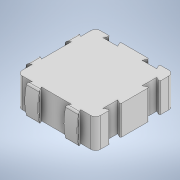
# Autodesk Inventor part: 2x2Base
Saved by Autodesk Inventor 2022.3 (Build 263350030, 350C)
## iProperties
Created: 2022-08-21
Part Number: 2x2Base
Material: Generic
Document SubType Name: Modeling
Designer: yiunf
Density: 1 g/cm^3
Appearance: Default
Author: yiunf
Autodesk Inventor part; units mm, degrees
ref_plane "YZ Plane" through (0, 0, 0) normal (1, 0, 0) x (0, 1, 0)
sketch "Sketch2" plane through (0, 0, 0) normal (0, 1, 0) x (-1, 0, 0)
  line L0 (-40, -40) -> (40, -40)
  line L1 (40, -40) -> (40, 40)
  line L2 (40, 40) -> (-40, 40)
  line L3 (-40, 40) -> (-40, -40)
  line L4 (-40, -40) -> (40, 40) construction
  line L5 (40, -40) -> (-40, 40) construction
  line L6 (0, 40) -> (40, 40)
  line L7 (20, 40) -> (20, 45)
  line L8 (20, 45) -> (27.5, 45)
  line L9 (20, 40) -> (25, 40)
  line L10 (25, 40) -> (27.5, 45)
  line L11 (20, 45) -> (12.5, 45)
  line L12 (20, 40) -> (15, 40)
  line L13 (15, 40) -> (12.5, 45)
  line L14 (20, 44.75) -> (27.0955, 44.75)
  line L15 (27.0955, 44.75) -> (24.8455, 40.25)
  line L16 (24.8455, 40.25) -> (20, 40.25)
  line L17 (20, 44.75) -> (12.9045, 44.75)
  line L18 (12.9045, 44.75) -> (15.1545, 40.25)
  line L19 (15.1545, 40.25) -> (20, 40.25)
  line L20 (20, 44.75) -> (20, 43.75)
  line L21 (20, 43.75) -> (26.875, 43.75)
  line L22 (20, 43.75) -> (13.125, 43.75)
  line L23 (40, 20) -> (45, 20)
  line L24 (45, 20) -> (45, 27.5)
  line L25 (40, 20) -> (40, 25)
  line L26 (40, 25) -> (45, 27.5)
  line L27 (40, 20) -> (40, 15)
  line L28 (40, 15) -> (45, 12.5)
  line L29 (45, 20) -> (45, 12.5)
  line L30 (44.75, 20) -> (44.75, 27.0955)
  line L31 (44.75, 27.0955) -> (40.25, 24.8455)
  line L32 (40.25, 24.8455) -> (40.25, 20)
  line L33 (44.75, 20) -> (44.75, 12.9045)
  line L34 (44.75, 12.9045) -> (40.25, 15.1545)
  line L35 (40.25, 15.1545) -> (40.25, 20)
  line L36 (44.75, 20) -> (43.75, 20)
  line L37 (43.75, 20) -> (43.75, 26.875)
  line L38 (43.75, 20) -> (43.75, 13.125)
  line L39 (-20, 40) -> (-20, 45)
  line L40 (-20, 44.75) -> (-20, 43.75)
  line L41 (-24.8455, 40.25) -> (-20, 40.25)
  line L42 (-20, 40) -> (-25, 40)
  line L43 (-27.0955, 44.75) -> (-24.8455, 40.25)
  line L44 (-25, 40) -> (-27.5, 45)
  line L45 (-20, 43.75) -> (-26.875, 43.75)
  line L46 (-20, 45) -> (-27.5, 45)
  line L47 (-20, 44.75) -> (-27.0955, 44.75)
  line L48 (-15.1545, 40.25) -> (-20, 40.25)
  line L49 (-20, 40) -> (-15, 40)
  line L50 (-20, 43.75) -> (-13.125, 43.75)
  line L51 (-20, 44.75) -> (-12.9045, 44.75)
  line L52 (-20, 45) -> (-12.5, 45)
  line L53 (-12.9045, 44.75) -> (-15.1545, 40.25)
  line L54 (-15, 40) -> (-12.5, 45)
  line L55 (40, -20) -> (40, -15)
  line L56 (44.75, -12.9045) -> (40.25, -15.1545)
  line L57 (40, -15) -> (45, -12.5)
  line L58 (43.75, -20) -> (43.75, -13.125)
  line L59 (44.75, -20) -> (44.75, -12.9045)
  line L60 (45, -20) -> (45, -12.5)
  line L61 (40.25, -15.1545) -> (40.25, -20)
  line L62 (40, -20) -> (45, -20)
  line L63 (40.25, -24.8455) -> (40.25, -20)
  line L64 (40, -20) -> (40, -25)
  line L65 (44.75, -27.0955) -> (40.25, -24.8455)
  line L66 (40, -25) -> (45, -27.5)
  line L67 (43.75, -20) -> (43.75, -26.875)
  line L68 (44.75, -20) -> (44.75, -27.0955)
  line L69 (45, -20) -> (45, -27.5)
  line L70 (44.75, -20) -> (43.75, -20)
  line L71 (20, -35) -> (27.5, -35)
  line L72 (25, -40) -> (27.5, -35)
  line L73 (20, -35) -> (12.5, -35)
  line L74 (15, -40) -> (12.5, -35)
  line L75 (-15, -40) -> (-12.5, -35)
  line L76 (-20, -35) -> (-12.5, -35)
  line L77 (-25, -40) -> (-27.5, -35)
  line L78 (-20, -35) -> (-27.5, -35)
  line L79 (24.8455, 40.25) -> (24.7205, 40)
  line L80 (15.1545, 40.25) -> (15.2795, 40)
  line L81 (-15.1545, 40.25) -> (-15.2795, 40)
  line L82 (-24.8455, 40.25) -> (-24.7205, 40)
  line L83 (40.25, 24.8455) -> (40, 24.7205)
  line L84 (40.25, 15.1545) -> (40, 15.2795)
  line L85 (40.25, -24.8455) -> (40, -24.7205)
  line L86 (40.25, -15.1545) -> (40, -15.2795)
  line L87 (-40, -25) -> (-35, -27.5)
  line L88 (-35, -20) -> (-35, -27.5)
  line L89 (-35, -20) -> (-35, -12.5)
  line L90 (-40, -15) -> (-35, -12.5)
  line L91 (-35, 20) -> (-35, 12.5)
  line L92 (-35, 20) -> (-35, 27.5)
  line L93 (-40, 15) -> (-35, 12.5)
  line L94 (-40, 25) -> (-35, 27.5)
  point P0 (0, 0)
  point P1 (26.875, -36.25)
  point P2 (13.125, -36.25)
  point P3 (-13.125, -36.25)
  point P4 (-26.875, -36.25)
  point P5 (-13.4045, 43.75)
  point P6 (-26.5955, 43.75)
  point P7 (43.75, -26.5955)
  point P8 (43.75, -13.4045)
  point P9 (43.75, 13.4045)
  point P10 (43.75, 26.5955)
  point P11 (26.5955, 43.75)
  point P12 (13.4045, 43.75)
  point P13 (-36.25, -26.875)
  point P14 (-36.25, -13.125)
  point P15 (-36.25, 13.125)
  point P16 (-36.25, 26.875)
  dimension "d0" = 80
  dimension "d1" = 80
  dimension "d2" = 5
  dimension "d3" = 7.5
  dimension "d4" = 5
  dimension "d5" = 0.25
  dimension "d6" = 0.25
  dimension "d7" = 1
  dimension "d10" = 40
  dimension "d17" = 40
  dimension "d24" = 80
  dimension "d51" = 80
  constraints: 190 end point, 34 point on line, 19 symmetric about line, 6 parallel, 4 horizontal, 4 midpoint, 3 perpendicular, 3 vertical, 1 collinear, 114 other
  measures "d0" distance of L2.end L1.end
  measures "d1" distance of L1.end L0.end
  measures "d2" distance of L7.start L7.end
  measures "d3" distance of L7.end L8.end
  measures "d4" distance of L7.start L9.end
  measures "d5" distance between parallel lines of L8 L14
  measures "d6" distance between parallel lines of L11 L17
  measures "d7" distance of L17.start L20.end
  measures "d10" distance of L7.start L39.start
  measures "d17" distance of L25.end L55.end
  measures "d24" distance of L7.end L71.start
  measures "d51" distance of L64.end L87.start
extrude "Extrusion1" add sketch "Sketch2" along normal blind 30 contours L3 L87 L88 L89 L90 L93 L91 L92 L94 L2 L1 L0 L72 L71 L73 L74 L75 L76 L78 L77 | L1 L62 L63 L85 | L82 L41 L39 L2 | L1 L86 L61 L62 | L63 L62 L67 L65 | L39 L48 L81 L2 | L43 L45 L39 L41 | L61 L56 L58 L62 | L39 L50 L53 L48 | L1 L23 L35 L84 | L1 L83 L32 L23 | L35 L23 L38 L34 | L80 L19 L7 L2 | L32 L31 L37 L23 | L7 L16 L79 L2 | L18 L22 L7 L19 | L7 L21 L15 L16
fillet "Fillet1" radius 1 8 edges at (-25, 15, -40) (-15, 15, -40) (15, 15, -40) (25, 15, -40) (40, 15, 15) (40, 15, 25) (40, 15, -15) (40, 15, -25)
fillet "Fillet2" radius 5 4 edges at (-40, 15, 40) (40, 15, 40) (40, 15, -40) (-40, 15, -40)
ref_plane "Work Plane1" through (-13.4045, 0, 43.75) normal (1, 0, 0) x (0, 1, 0)
sketch "Sketch3" plane through (-13.4045, 0, 43.75) normal (1, 0, 0) x (0, 1, 0)
  line L0 (0, -3.75) -> (30, -3.75) projected
  line L1 (15, -3.75) -> (15, 2)
  line L2 (15, 2) -> (15, 1)
  line L3 (30, -3.75) -> (30, 0) projected
  arc A0 (30, 0) -> (0, 0) centre (15, -55.25) ccw
  line L4 (30, 0) -> (25, 0)
  line L5 (0, 0) -> (30, 0) projected
  line L6 (25, 0) -> (5, 0)
  arc A1 (25, 0) -> (5, 0) centre (15, -49.5) ccw
  point P0 (0, -43.75)
  dimension "d34" = 5.75
  dimension "d35" = 1
  dimension "d36" = 5
  dimension "d37" = 20
  constraints: 8 end point, 6 point on circle, 3 point on line, 2 centre point, 1 midpoint, 1 vertical
  measures "d34" distance of L1.start L1.end
  measures "d35" distance of L1.end L2.end
  measures "d36" distance of L3.end L4.end
  measures "d37" distance of L4.end L6.end
extrude "Extrusion2" add sketch "Sketch3" against normal blind 13.191 contours L4 A1 L1 A0 | A1 L5 A0 L1
sketch "Sketch4" plane through (0, 30, 0) normal (0, 1, 0) x (1, 0, 0)
  line L0 (-26.5955, -43.75) -> (-13.4045, -43.75) projected
  line L1 (-20, -43.75) -> (-20, 0)
  line L2 (-20, 0) -> (-43.75, -20)
  line L3 (-43.75, -13.4045) -> (-43.75, -26.5955) projected
  line L4 (-43.75, -20) -> (-20, -20)
  point P0 (0, 0)
  constraints: 6 end point, 2 midpoint, 1 perpendicular, 1 point on line, 1 vertical
pattern_circular "Circular Pattern1" count 2 over 270 about axis through (-20, 30, 20) along (0, 1, 0) of "Extrusion2"
pattern_linear "Rectangular Pattern1" count 2 spacing 40 along (1, 0, 0) of "Extrusion2"
ref_plane "Work Plane2" through (-43.75, 0, -26.5955) normal (0, 0, 1) x (0, 1, 0)
sketch "Sketch5" plane through (-43.75, 0, -26.5955) normal (0, 0, 1) x (0, 1, 0)
  line L0 (30, 0) -> (30, -3.75) projected
  line L1 (0, 0) -> (30, 0) projected
  arc A0 (30, 0) -> (0, 0) centre (15, -55.25) ccw
  arc A1 (25, 0) -> (5, 0) centre (15, -49.5) ccw projected
  arc A2 (25, 0) -> (5, 0) centre (15, -49.5) ccw
  point P0 (0, -43.75)
  constraints: 4 point on circle, 2 centre point
extrude "Extrusion3" add sketch "Sketch5" along normal blind 13.191 contours A0 L1 A1
fillet "Fillet3" radius 2 8 edges at (-26.5955, 30, 43.75) (-20, 0, 43.75) (20, 30, 43.75) (20, 0, 43.75) (-43.75, 30, 20) (-43.75, 30, -13.4045) (-43.75, 0, -13.4045) (-43.75, 0, 20)
body "Solid1"
